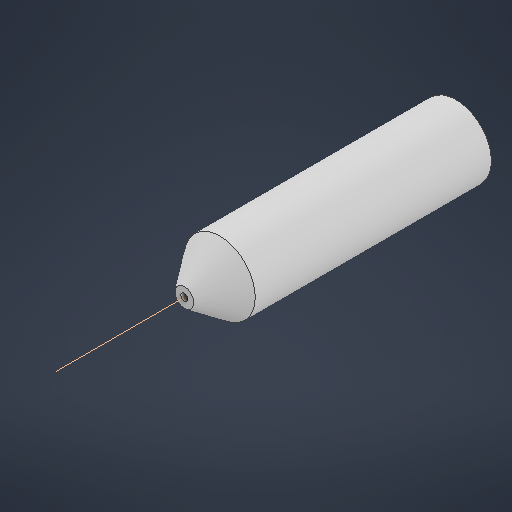
# Autodesk Inventor part: Nozzle
Saved by Autodesk Inventor 2025.3 (Build 293356030, 356C)
## iProperties
Created: 2025-09-18
Part Number: Nozzle
Material: Generic
Document SubType Name: Modeling
Designer: yo
Density: 1 g/cm^3
Appearance: Default
Author: yo
Autodesk Inventor part; units mm, degrees
ref_plane "YZ Plane" through (0, 0, 0) normal (1, 0, 0) x (0, 1, 0)
ref_plane "XZ Plane" through (0, 0, 0) normal (0, 1, 0) x (-1, 0, 0)
ref_plane "XY Plane" through (0, 0, 0) normal (0, 0, 1) x (1, 0, 0)
sketch "Sketch1" plane through (0, 0, 0) normal (0, 0, 1) x (1, 0, 0)
  circle A0 centre (0, 0) radius 3
  circle A1 centre (0, 0) radius 2
  dimension "d0" = 6
  dimension "d1" = 4
  constraints: 2 centre point, 2 coincident
  measures "d0" diameter of A0
  measures "d1" diameter of A1
extrude "Extrusion1" add sketch "Sketch1" along normal mid plane 20
sketch "Sketch2" plane through (0, 0, 0) normal (1, 0, 0) x (0, 1, 0)
  line L0 (3, 10) -> (-3, 10) construction
  line L1 (0, 10) -> (0, 13) construction
  line L2 (-3, -10) -> (-3, 10) construction
  line L3 (-3, 10) -> (-0.8, 13)
  line L4 (-0.8, 13) -> (-0.3, 13)
  line L5 (-0.3, 13) -> (-2.5, 10)
  line L6 (-3, 10) -> (-2.5, 10)
  point P0 (0, 0)
  point P1 (-0.55, 13)
  dimension "d4" = 3
  dimension "d6" = 0.3
  dimension "d7" = 0.5
  constraints: 10 end point, 2 midpoint, 1 collinear, 1 horizontal, 1 horizontal alignment, 1 parallel, 1 point on line, 1 vertical
  measures "d4" distance of L1.start L1.end
  measures "d6" distance of L4.end L1.end
  measures "d7" distance of L3.end L4.end
revolve "Revolution1" add sketch "Sketch2" angle 360 about axis through (0, 0, 10) along (0, 0, 1)
body "Solid1"
